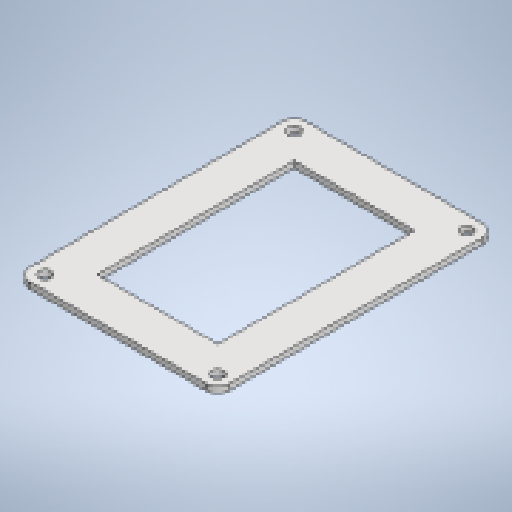
# Autodesk Inventor part: PRS 940-51 FDS Diam way flange 1
Saved by Autodesk Inventor 2025.3 (Build 293356030, 356C)
## iProperties
Created: 2025-06-24
Part Number: PRS 940-51 FDS Diam way flange 1
Material: Stainless Steel
Document SubType Name: Sheet Metal
Designer: admin
Mass: 205.824 g
Surface Area: 199.633 cm^2
Volume: 25.728 cm^3
Density: 8 g/cm^3
Flat Pattern Width: 10 cm
Flat Pattern Length: 13.8 cm
Flat Pattern Area: 138 cm^2
Sheet Metal Rule: AISI304 2mm Die16
Sheet Metal Width: 100,000 mm
Sheet Metal Length: 138,000 mm
Sheet Metal Area: 13800,000 mm^2
Appearance: Default
Author: user
Autodesk Inventor part; units mm, degrees
ref_plane "YZ Plane" through (0, 0, 0) normal (1, 0, 0) x (0, 1, 0)
ref_plane "XZ Plane" through (0, 0, 0) normal (0, 1, 0) x (-1, 0, 0)
ref_plane "XY Plane" through (0, 0, 0) normal (0, 0, 1) x (1, 0, 0)
sketch "Sketch1" plane through (0, 0, 0) normal (0, 0, 1) x (1, 0, 0)
  line L0 (-50, -69) -> (50, -69)
  line L1 (50, -69) -> (50, 69)
  line L2 (50, 69) -> (-50, 69)
  line L3 (-50, 69) -> (-50, -69)
  line L4 (-50, -69) -> (50, 69) construction
  line L5 (50, -69) -> (-50, 69) construction
  line L6 (30, -49) -> (-30, -49)
  line L7 (-30, -49) -> (-30, 49)
  line L8 (-30, 49) -> (30, 49)
  line L9 (30, 49) -> (30, -49)
  line L10 (30, -49) -> (-30, 49) construction
  line L11 (-30, -49) -> (30, 49) construction
  point P0 (0, 0)
  dimension "d172" = 60
  dimension "d180" = 20
  dimension "d181" = 20
  dimension "d182" = 98
  measures "d172" distance of L7.end L8.end
  measures "d180" distance between parallel lines of L3 L7
  measures "d181" distance between parallel lines of L8 L2
  measures "d182" distance of L6.end L7.end
extrude "Plate5" add sketch "Sketch1" along normal blind 3
sketch "Sketch9" plane through (0, 0, 3) normal (0, 0, 1) x (1, 0, 0)
  circle A0 centre (43, -62) radius 3
  line L0 (43, 62) -> (-43, 62) construction
  line L1 (-43, 62) -> (-43, -62) construction
  line L2 (-43, -62) -> (43, -62) construction
  line L3 (43, -62) -> (43, 62) construction
  line L4 (43, 62) -> (-43, -62) construction
  line L5 (-43, 62) -> (43, -62) construction
  circle A1 centre (-43, -62) radius 3
  circle A2 centre (43, 62) radius 3
  circle A3 centre (-43, 62) radius 3
  line L6 (-30, -49) -> (-30, 49) projected
  line L7 (-30, 49) -> (30, 49) projected
  line L8 (30, 49) -> (30, -49) projected
  line L9 (30, -49) -> (-30, -49) projected
  line L10 (50, -69) -> (-50, -69) projected
  line L11 (50, 69) -> (50, -69) projected
  line L12 (-50, 69) -> (50, 69) projected
  line L13 (-50, -69) -> (-50, 69) projected
  circle A4 centre (-43, 0) radius 3 construction
  circle A5 centre (43, 0) radius 3 construction
  point P0 (0, 0)
  dimension "d174" = 6
  dimension "d183" = 7
  dimension "d184" = 7
  constraints: 12 end point, 7 coincident, 6 centre point, 5 equal radius, 4 midpoint, 2 parallel, 1 horizontal, 1 perpendicular
  measures "d174" diameter of A0
  measures "d183" distance from line of L0.start L12
  measures "d184" distance from line of L0.start L11
extrude "Cut2" cut sketch "Sketch9" against normal blind 3 contours A0 | A1 | A2 | A3
fillet "Corner Round1" radius 6 4 edges at (50, 69, 1.5) (-50, 69, 1.5) (-50, -69, 1.5) (50, -69, 1.5)
body "Solid3"
